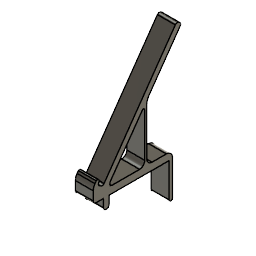
display-holder (Autodesk Fusion 360 design; units mm, degrees)
Autodesk Fusion 360 part; units mm, degrees
note: some values were not read from the file. Set by a fixed rule: which sketch regions a step uses.
(part 1 of 3)
sketch "Sketch1" plane through (0, 0, 0) normal (0, 1, 0) x (1, 0, 0) in component "breadboard"
  line L0 (0, 0) -> (83, 0)
  line L1 (83, 0) -> (83, -10)
  line L2 (83, -10) -> (0, -10)
  line L3 (0, -10) -> (0, 0)
  line L4 (13, 0) -> (17, 0)
  line L5 (17, 0) -> (17, -5)
  line L6 (17, -5) -> (13, -5)
  line L7 (13, -5) -> (13, 0)
  line L8 (66, 0) -> (70, 0)
  line L9 (70, 0) -> (70, -5)
  line L10 (70, -5) -> (66, -5)
  line L11 (66, -5) -> (66, 0)
  dimension "d1" = 10
  dimension "d2" = 83
  constraint horizontal L0
  constraint vertical L1
  constraint horizontal L2
  constraint vertical L3
  constraint coincident L0.start L3.end
  constraint horizontal L4
  constraint vertical L5
  constraint horizontal L6
  constraint vertical L7
  constraint horizontal L8
  constraint vertical L9
  constraint horizontal L10
  constraint vertical L11
  measures "d1" distance of L0.start L2.end
  measures "d2" distance of L0.start L0.end
extrude "Extrude3" add sketch "Sketch1" along normal blind 10 makes body 1 in component "breadboard"
extrude "Extrude5" add sketch "Sketch1" against normal blind 1 contours L0 L4 L5 L6 L7 | L0 L8 L9 L10 L11 bodies 1 in component "breadboard"
sketch "Sketch5" plane through (83, 0, 0) normal (1, 0, 0) x (0, 1, 0) in component "breadboard"
  line L0 (0, 10) -> (0, 0)
  line L1 (0, 0) -> (10, 0)
  line L2 (10, 0) -> (10, 10)
  line L3 (10, 10) -> (0, 10)
  line L4 (3, 0) -> (7, 0)
  line L5 (7, 0) -> (7, 5)
  line L6 (7, 5) -> (3, 5)
  line L7 (3, 5) -> (3, 0)
  constraint coincident L1 L4.start
  constraint horizontal L4
  constraint vertical L5
  constraint horizontal L6
  constraint vertical L7
extrude "Extrude6" add sketch "Sketch5" along normal blind 1 contours L1 L4 L5 L6 L7 bodies 1 in component "breadboard"
sketch "Sketch6" plane through (0, 0, 0) normal (-1, 0, 0) x (0, -1, 0) in component "breadboard"
  line L0 (0, 0) -> (0, 10)
  line L1 (0, 10) -> (-10, 10)
  line L2 (-10, 10) -> (-10, 0)
  line L3 (-10, 0) -> (0, 0)
  line L4 (-7, 0) -> (-3, 0)
  line L5 (-3, 0) -> (-3, 4)
  line L6 (-3, 4) -> (-7, 4)
  line L7 (-7, 4) -> (-7, 0)
  line L8 (-3, 5) -> (-3, 0)
  point P0 (-7, 0)
  constraint coincident P0 L4.start
  constraint horizontal L4
  constraint vertical L5
  constraint horizontal L6
  constraint vertical L7
  constraint coincident L5.end L8
extrude "Extrude7" cut sketch "Sketch6" against normal blind 1 contours L3 L4 L5 L6 L7 L8 bodies 1 in component "breadboard"
sketch "Sketch8" plane through (0, 0, 0) normal (0, 0, 1) x (1, 0, 0) in component "breadboard"
  line L0 (0, 45) -> (83, 45)
  line L1 (83, 45) -> (83, 10)
  line L2 (83, 10) -> (0, 10)
  line L3 (0, 10) -> (0, 45)
  point P0 (0, 45)
  point P1 (83, 10)
  constraint horizontal L0
  constraint vertical L1
  constraint horizontal L2
  constraint vertical L3
  constraint coincident P1 L1.end
  constraint coincident P0 L0.start
extrude "Extrude8" add sketch "Sketch8" along normal blind 10 separate body makes body 2 in component "breadboard"
sketch "Sketch9" plane through (0, 0, 10) normal (0, 0, 1) x (-1, 0, 0) in component "breadboard"
  line L0 (-83, -10) -> (-83, -45)
  line L1 (0, -45) -> (0, -10)
  line L2 (0, -26.5) -> (-83, -26.5)
  line L3 (0, -28.5) -> (-83, -28.5)
  line L4 (0, -10) -> (-83, -10)
  line L5 (-83, -45) -> (0, -45)
  line L6 (-5.0001, -15.25) -> (-5.0001, -17.25)
  line L7 (-5.0001, -17.25) -> (-3.0001, -17.25)
  line L8 (-3.0001, -17.25) -> (-3.0001, -15.25)
  line L9 (-3.0001, -15.25) -> (-5.0001, -15.25)
  line L10 (-3.0001, -17.75) -> (-5.0001, -17.75)
  line L11 (-5.0001, -17.75) -> (-5.0001, -19.75)
  line L12 (-5.0001, -19.75) -> (-3.0001, -19.75)
  line L13 (-3.0001, -19.75) -> (-3.0001, -17.75)
  line L14 (-5.0001, -22.25) -> (-3.0001, -22.25)
  line L15 (-3.0001, -22.25) -> (-3.0001, -20.25)
  line L16 (-3.0001, -20.25) -> (-5.0001, -20.25)
  line L17 (-5.0001, -20.25) -> (-5.0001, -22.25)
  line L18 (-5.0001, -24.75) -> (-3.0001, -24.75)
  line L19 (-3.0001, -24.75) -> (-3.0001, -22.75)
  line L20 (-5.0001, -22.75) -> (-5.0001, -24.75)
  line L21 (-3.0001, -22.75) -> (-5.0001, -22.75)
  line L22 (-5.0001, -14.75) -> (-3.0001, -14.75)
  line L23 (-3.0001, -14.75) -> (-3.0001, -12.75)
  line L24 (-3.0001, -12.75) -> (-5.0001, -12.75)
  line L25 (-5.0001, -12.75) -> (-5.0001, -14.75)
  line L26 (-7.5001, -15.25) -> (-7.5001, -17.25)
  line L27 (-5.5001, -24.75) -> (-5.5001, -22.75)
  line L28 (-5.5001, -22.75) -> (-7.5001, -22.75)
  line L29 (-5.5001, -17.25) -> (-5.5001, -15.25)
  line L30 (-7.5001, -14.75) -> (-5.5001, -14.75)
  line L31 (-7.5001, -12.75) -> (-7.5001, -14.75)
  line L32 (-5.5001, -15.25) -> (-7.5001, -15.25)
  line L33 (-7.5001, -17.25) -> (-5.5001, -17.25)
  line L34 (-7.5001, -22.75) -> (-7.5001, -24.75)
  line L35 (-5.5001, -22.25) -> (-5.5001, -20.25)
  line L36 (-5.5001, -12.75) -> (-7.5001, -12.75)
  line L37 (-5.5001, -20.25) -> (-7.5001, -20.25)
  line L38 (-7.5001, -22.25) -> (-5.5001, -22.25)
  line L39 (-5.5001, -17.75) -> (-7.5001, -17.75)
  line L40 (-5.5001, -19.75) -> (-5.5001, -17.75)
  line L41 (-7.5001, -19.75) -> (-5.5001, -19.75)
  line L42 (-7.5001, -20.25) -> (-7.5001, -22.25)
  line L43 (-7.5001, -17.75) -> (-7.5001, -19.75)
  line L44 (-5.5001, -14.75) -> (-5.5001, -12.75)
  line L45 (-7.5001, -24.75) -> (-5.5001, -24.75)
  line L46 (-12.5001, -15.25) -> (-12.5001, -17.25)
  line L47 (-8.0001, -22.25) -> (-8.0001, -20.25)
  line L48 (-10.5001, -22.25) -> (-10.5001, -20.25)
  line L49 (-10.5001, -15.25) -> (-12.5001, -15.25)
  line L50 (-10.5001, -20.25) -> (-12.5001, -20.25)
  line L51 (-8.0001, -20.25) -> (-10.0001, -20.25)
  line L52 (-10.5001, -14.75) -> (-10.5001, -12.75)
  line L53 (-12.5001, -12.75) -> (-12.5001, -14.75)
  line L54 (-12.5001, -20.25) -> (-12.5001, -22.25)
  line L55 (-8.0001, -12.75) -> (-10.0001, -12.75)
  line L56 (-10.5001, -19.75) -> (-10.5001, -17.75)
  line L57 (-10.5001, -17.25) -> (-10.5001, -15.25)
  line L58 (-10.0001, -22.25) -> (-8.0001, -22.25)
  line L59 (-12.5001, -19.75) -> (-10.5001, -19.75)
  line L60 (-8.0001, -15.25) -> (-10.0001, -15.25)
  line L61 (-10.0001, -15.25) -> (-10.0001, -17.25)
  line L62 (-8.0001, -22.75) -> (-10.0001, -22.75)
  line L63 (-10.0001, -24.75) -> (-8.0001, -24.75)
  line L64 (-8.0001, -19.75) -> (-8.0001, -17.75)
  line L65 (-10.0001, -20.25) -> (-10.0001, -22.25)
  line L66 (-8.0001, -17.75) -> (-10.0001, -17.75)
  line L67 (-12.5001, -17.75) -> (-12.5001, -19.75)
  line L68 (-10.0001, -22.75) -> (-10.0001, -24.75)
  line L69 (-10.5001, -17.75) -> (-12.5001, -17.75)
  line L70 (-10.5001, -12.75) -> (-12.5001, -12.75)
  line L71 (-8.0001, -24.75) -> (-8.0001, -22.75)
  line L72 (-10.0001, -17.75) -> (-10.0001, -19.75)
  line L73 (-10.0001, -12.75) -> (-10.0001, -14.75)
  line L74 (-12.5001, -14.75) -> (-10.5001, -14.75)
  line L75 (-12.5001, -24.75) -> (-10.5001, -24.75)
  line L76 (-12.5001, -22.25) -> (-10.5001, -22.25)
  line L77 (-10.5001, -22.75) -> (-12.5001, -22.75)
  line L78 (-10.0001, -14.75) -> (-8.0001, -14.75)
  line L79 (-8.0001, -14.75) -> (-8.0001, -12.75)
  line L80 (-12.5001, -17.25) -> (-10.5001, -17.25)
  line L81 (-8.0001, -17.25) -> (-8.0001, -15.25)
  line L82 (-10.5001, -24.75) -> (-10.5001, -22.75)
  line L83 (-12.5001, -22.75) -> (-12.5001, -24.75)
  line L84 (-10.0001, -17.25) -> (-8.0001, -17.25)
  line L85 (-10.0001, -19.75) -> (-8.0001, -19.75)
  line L86 (-13.0001, -17.25) -> (-13.0001, -15.25)
  line L87 (-17.5001, -17.75) -> (-17.5001, -19.75)
  line L88 (-15.0001, -12.75) -> (-15.0001, -14.75)
  line L89 (-13.0001, -15.25) -> (-15.0001, -15.25)
  line L90 (-15.5001, -17.25) -> (-15.5001, -15.25)
  line L91 (-15.0001, -22.25) -> (-13.0001, -22.25)
  line L92 (-15.5001, -24.75) -> (-15.5001, -22.75)
  line L93 (-18.0001, -19.75) -> (-18.0001, -17.75)
  line L94 (-15.5001, -22.75) -> (-17.5001, -22.75)
  line L95 (-13.0001, -22.75) -> (-15.0001, -22.75)
  line L96 (-13.0001, -14.75) -> (-13.0001, -12.75)
  line L97 (-15.5001, -14.75) -> (-15.5001, -12.75)
  line L98 (-15.5001, -19.75) -> (-15.5001, -17.75)
  line L99 (-15.0001, -14.75) -> (-13.0001, -14.75)
  line L100 (-13.0001, -24.75) -> (-13.0001, -22.75)
  line L101 (-13.0001, -12.75) -> (-15.0001, -12.75)
  line L102 (-15.0001, -17.25) -> (-13.0001, -17.25)
  line L103 (-15.0001, -24.75) -> (-13.0001, -24.75)
  line L104 (-17.5001, -20.25) -> (-17.5001, -22.25)
  line L105 (-18.0001, -15.25) -> (-20.0001, -15.25)
  line L106 (-18.0001, -12.75) -> (-20.0001, -12.75)
  line L107 (-17.5001, -12.75) -> (-17.5001, -14.75)
  line L108 (-15.0001, -20.25) -> (-15.0001, -22.25)
  line L109 (-15.0001, -19.75) -> (-13.0001, -19.75)
  line L110 (-18.0001, -17.25) -> (-18.0001, -15.25)
  line L111 (-20.0001, -14.75) -> (-18.0001, -14.75)
  line L112 (-22.5001, -20.25) -> (-22.5001, -22.25)
  line L113 (-20.0001, -12.75) -> (-20.0001, -14.75)
  line L114 (-18.0001, -14.75) -> (-18.0001, -12.75)
  line L115 (-20.5001, -20.25) -> (-22.5001, -20.25)
  line L116 (-20.5001, -22.75) -> (-22.5001, -22.75)
  line L117 (-22.5001, -12.75) -> (-22.5001, -14.75)
  line L118 (-20.5001, -17.25) -> (-20.5001, -15.25)
  line L119 (-20.0001, -15.25) -> (-20.0001, -17.25)
  line L120 (-20.5001, -15.25) -> (-22.5001, -15.25)
  line L121 (-22.5001, -15.25) -> (-22.5001, -17.25)
  line L122 (-17.5001, -15.25) -> (-17.5001, -17.25)
  line L123 (-15.5001, -22.25) -> (-15.5001, -20.25)
  line L124 (-20.0001, -20.25) -> (-20.0001, -22.25)
  line L125 (-18.0001, -22.25) -> (-18.0001, -20.25)
  line L126 (-13.0001, -22.25) -> (-13.0001, -20.25)
  line L127 (-22.5001, -19.75) -> (-20.5001, -19.75)
  line L128 (-22.5001, -17.25) -> (-20.5001, -17.25)
  line L129 (-22.5001, -14.75) -> (-20.5001, -14.75)
  line L130 (-20.5001, -12.75) -> (-22.5001, -12.75)
  line L131 (-20.0001, -17.25) -> (-18.0001, -17.25)
  line L132 (-20.0001, -17.75) -> (-20.0001, -19.75)
  line L133 (-15.5001, -20.25) -> (-17.5001, -20.25)
  line L134 (-15.5001, -12.75) -> (-17.5001, -12.75)
  line L135 (-20.0001, -22.75) -> (-20.0001, -24.75)
  line L136 (-20.5001, -17.75) -> (-22.5001, -17.75)
  line L137 (-20.0001, -24.75) -> (-18.0001, -24.75)
  line L138 (-22.5001, -17.75) -> (-22.5001, -19.75)
  line L139 (-18.0001, -22.75) -> (-20.0001, -22.75)
  line L140 (-20.0001, -22.25) -> (-18.0001, -22.25)
  line L141 (-20.5001, -19.75) -> (-20.5001, -17.75)
  line L142 (-18.0001, -24.75) -> (-18.0001, -22.75)
  line L143 (-17.5001, -22.75) -> (-17.5001, -24.75)
  line L144 (-20.5001, -14.75) -> (-20.5001, -12.75)
  line L145 (-13.0001, -20.25) -> (-15.0001, -20.25)
  line L146 (-13.0001, -19.75) -> (-13.0001, -17.75)
  line L147 (-17.5001, -17.25) -> (-15.5001, -17.25)
  line L148 (-17.5001, -19.75) -> (-15.5001, -19.75)
  line L149 (-18.0001, -20.25) -> (-20.0001, -20.25)
  line L150 (-15.5001, -17.75) -> (-17.5001, -17.75)
  line L151 (-15.0001, -15.25) -> (-15.0001, -17.25)
  line L152 (-15.0001, -22.75) -> (-15.0001, -24.75)
  line L153 (-17.5001, -14.75) -> (-15.5001, -14.75)
  line L154 (-18.0001, -17.75) -> (-20.0001, -17.75)
  line L155 (-13.0001, -17.75) -> (-15.0001, -17.75)
  line L156 (-15.5001, -15.25) -> (-17.5001, -15.25)
  line L157 (-22.5001, -22.25) -> (-20.5001, -22.25)
  line L158 (-22.5001, -22.75) -> (-22.5001, -24.75)
  line L159 (-20.5001, -22.25) -> (-20.5001, -20.25)
  line L160 (-17.5001, -24.75) -> (-15.5001, -24.75)
  line L161 (-20.5001, -24.75) -> (-20.5001, -22.75)
  line L162 (-20.0001, -19.75) -> (-18.0001, -19.75)
  line L163 (-17.5001, -22.25) -> (-15.5001, -22.25)
  line L164 (-15.0001, -17.75) -> (-15.0001, -19.75)
  line L165 (-22.5001, -24.75) -> (-20.5001, -24.75)
  line L166 (-40.5001, -19.75) -> (-40.5001, -17.75)
  line L167 (-38.0001, -20.25) -> (-40.0001, -20.25)
  line L168 (-42.5001, -17.25) -> (-40.5001, -17.25)
  line L169 (-37.5001, -17.75) -> (-37.5001, -19.75)
  line L170 (-40.5001, -17.75) -> (-42.5001, -17.75)
  line L171 (-40.0001, -17.75) -> (-40.0001, -19.75)
  line L172 (-40.5001, -20.25) -> (-42.5001, -20.25)
  line L173 (-40.0001, -17.25) -> (-38.0001, -17.25)
  line L174 (-40.0001, -19.75) -> (-38.0001, -19.75)
  line L175 (-35.5001, -17.75) -> (-37.5001, -17.75)
  line L176 (-35.5001, -20.25) -> (-37.5001, -20.25)
  line L177 (-37.5001, -19.75) -> (-35.5001, -19.75)
  line L178 (-37.5001, -17.25) -> (-35.5001, -17.25)
  line L179 (-42.5001, -19.75) -> (-40.5001, -19.75)
  line L180 (-38.0001, -17.75) -> (-40.0001, -17.75)
  line L181 (-35.5001, -19.75) -> (-35.5001, -17.75)
  line L182 (-38.0001, -19.75) -> (-38.0001, -17.75)
  line L183 (-42.5001, -17.75) -> (-42.5001, -19.75)
  line L184 (-42.5001, -22.75) -> (-42.5001, -24.75)
  line L185 (-38.0001, -22.75) -> (-40.0001, -22.75)
  line L186 (-35.5001, -22.25) -> (-35.5001, -20.25)
  line L187 (-27.5001, -20.25) -> (-27.5001, -22.25)
  line L188 (-35.5001, -12.75) -> (-37.5001, -12.75)
  line L189 (-40.0001, -20.25) -> (-40.0001, -22.25)
  line L190 (-42.5001, -22.25) -> (-40.5001, -22.25)
  line L191 (-37.5001, -14.75) -> (-35.5001, -14.75)
  line L192 (-35.5001, -22.75) -> (-37.5001, -22.75)
  line L193 (-40.5001, -12.75) -> (-42.5001, -12.75)
  line L194 (-25.0001, -17.25) -> (-23.0001, -17.25)
  line L195 (-37.5001, -24.75) -> (-35.5001, -24.75)
  line L196 (-37.5001, -20.25) -> (-37.5001, -22.25)
  line L197 (-25.0001, -24.75) -> (-23.0001, -24.75)
  line L198 (-35.5001, -15.25) -> (-37.5001, -15.25)
  line L199 (-38.0001, -24.75) -> (-38.0001, -22.75)
  line L200 (-40.0001, -22.25) -> (-38.0001, -22.25)
  line L201 (-42.5001, -24.75) -> (-40.5001, -24.75)
  line L202 (-42.5001, -20.25) -> (-42.5001, -22.25)
  line L203 (-40.5001, -15.25) -> (-42.5001, -15.25)
  line L204 (-40.0001, -24.75) -> (-38.0001, -24.75)
  line L205 (-40.5001, -24.75) -> (-40.5001, -22.75)
  line L206 (-38.0001, -22.25) -> (-38.0001, -20.25)
  line L207 (-42.5001, -14.75) -> (-40.5001, -14.75)
  line L208 (-40.0001, -15.25) -> (-40.0001, -17.25)
  line L209 (-38.0001, -17.25) -> (-38.0001, -15.25)
  line L210 (-37.5001, -22.75) -> (-37.5001, -24.75)
  line L211 (-40.5001, -22.75) -> (-42.5001, -22.75)
  line L212 (-40.5001, -17.25) -> (-40.5001, -15.25)
  line L213 (-37.5001, -22.25) -> (-35.5001, -22.25)
  line L214 (-25.0001, -19.75) -> (-23.0001, -19.75)
  line L215 (-42.5001, -15.25) -> (-42.5001, -17.25)
  line L216 (-32.5001, -20.25) -> (-32.5001, -22.25)
  line L217 (-37.5001, -15.25) -> (-37.5001, -17.25)
  line L218 (-40.5001, -22.25) -> (-40.5001, -20.25)
  line L219 (-40.0001, -22.75) -> (-40.0001, -24.75)
  line L220 (-32.5001, -17.75) -> (-32.5001, -19.75)
  line L221 (-35.0001, -17.75) -> (-35.0001, -19.75)
  line L222 (-28.0001, -22.75) -> (-30.0001, -22.75)
  line L223 (-40.0001, -14.75) -> (-38.0001, -14.75)
  line L224 (-38.0001, -15.25) -> (-40.0001, -15.25)
  line L225 (-27.5001, -17.75) -> (-27.5001, -19.75)
  line L226 (-27.5001, -24.75) -> (-25.5001, -24.75)
  line L227 (-32.5001, -15.25) -> (-32.5001, -17.25)
  line L228 (-33.0001, -20.25) -> (-35.0001, -20.25)
  line L229 (-35.0001, -17.25) -> (-33.0001, -17.25)
  line L230 (-25.5001, -15.25) -> (-27.5001, -15.25)
  line L231 (-27.5001, -22.75) -> (-27.5001, -24.75)
  line L232 (-35.5001, -24.75) -> (-35.5001, -22.75)
  line L233 (-25.0001, -20.25) -> (-25.0001, -22.25)
  line L234 (-35.0001, -19.75) -> (-33.0001, -19.75)
  line L235 (-40.5001, -14.75) -> (-40.5001, -12.75)
  line L236 (-30.5001, -17.25) -> (-30.5001, -15.25)
  line L237 (-30.0001, -17.75) -> (-30.0001, -19.75)
  line L238 (-30.0001, -22.75) -> (-30.0001, -24.75)
  line L239 (-25.5001, -22.75) -> (-27.5001, -22.75)
  line L240 (-28.0001, -19.75) -> (-28.0001, -17.75)
  line L241 (-30.0001, -20.25) -> (-30.0001, -22.25)
  line L242 (-37.5001, -12.75) -> (-37.5001, -14.75)
  line L243 (-30.5001, -20.25) -> (-32.5001, -20.25)
  line L244 (-27.5001, -17.25) -> (-25.5001, -17.25)
  line L245 (-32.5001, -24.75) -> (-30.5001, -24.75)
  line L246 (-25.5001, -12.75) -> (-27.5001, -12.75)
  line L247 (-25.0001, -17.75) -> (-25.0001, -19.75)
  line L248 (-23.0001, -22.25) -> (-23.0001, -20.25)
  line L249 (-32.5001, -22.25) -> (-30.5001, -22.25)
  line L250 (-30.5001, -19.75) -> (-30.5001, -17.75)
  line L251 (-28.0001, -20.25) -> (-30.0001, -20.25)
  line L252 (-32.5001, -19.75) -> (-30.5001, -19.75)
  line L253 (-35.0001, -15.25) -> (-35.0001, -17.25)
  line L254 (-35.5001, -17.25) -> (-35.5001, -15.25)
  line L255 (-33.0001, -17.25) -> (-33.0001, -15.25)
  line L256 (-42.5001, -12.75) -> (-42.5001, -14.75)
  line L257 (-38.0001, -12.75) -> (-40.0001, -12.75)
  line L258 (-30.5001, -17.75) -> (-32.5001, -17.75)
  line L259 (-25.5001, -22.25) -> (-25.5001, -20.25)
  line L260 (-33.0001, -19.75) -> (-33.0001, -17.75)
  line L261 (-30.0001, -22.25) -> (-28.0001, -22.25)
  line L262 (-30.0001, -19.75) -> (-28.0001, -19.75)
  line L263 (-28.0001, -24.75) -> (-28.0001, -22.75)
  line L264 (-30.0001, -24.75) -> (-28.0001, -24.75)
  line L265 (-25.5001, -17.75) -> (-27.5001, -17.75)
  line L266 (-23.0001, -20.25) -> (-25.0001, -20.25)
  line L267 (-33.0001, -17.75) -> (-35.0001, -17.75)
  line L268 (-32.5001, -22.75) -> (-32.5001, -24.75)
  line L269 (-28.0001, -22.25) -> (-28.0001, -20.25)
  line L270 (-27.5001, -22.25) -> (-25.5001, -22.25)
  line L271 (-30.5001, -22.75) -> (-32.5001, -22.75)
  line L272 (-40.0001, -12.75) -> (-40.0001, -14.75)
  line L273 (-38.0001, -14.75) -> (-38.0001, -12.75)
  line L274 (-28.0001, -17.75) -> (-30.0001, -17.75)
  line L275 (-30.5001, -12.75) -> (-32.5001, -12.75)
  line L276 (-30.5001, -14.75) -> (-30.5001, -12.75)
  line L277 (-30.5001, -15.25) -> (-32.5001, -15.25)
  line L278 (-27.5001, -12.75) -> (-27.5001, -14.75)
  line L279 (-33.0001, -15.25) -> (-35.0001, -15.25)
  line L280 (-30.0001, -17.25) -> (-28.0001, -17.25)
  line L281 (-30.0001, -15.25) -> (-30.0001, -17.25)
  line L282 (-27.5001, -15.25) -> (-27.5001, -17.25)
  line L283 (-25.0001, -22.25) -> (-23.0001, -22.25)
  line L284 (-23.0001, -19.75) -> (-23.0001, -17.75)
  line L285 (-33.0001, -12.75) -> (-35.0001, -12.75)
  line L286 (-35.0001, -12.75) -> (-35.0001, -14.75)
  line L287 (-28.0001, -12.75) -> (-30.0001, -12.75)
  line L288 (-25.5001, -24.75) -> (-25.5001, -22.75)
  line L289 (-27.5001, -14.75) -> (-25.5001, -14.75)
  line L290 (-25.0001, -22.75) -> (-25.0001, -24.75)
  line L291 (-28.0001, -17.25) -> (-28.0001, -15.25)
  line L292 (-35.0001, -14.75) -> (-33.0001, -14.75)
  line L293 (-25.5001, -19.75) -> (-25.5001, -17.75)
  line L294 (-30.0001, -14.75) -> (-28.0001, -14.75)
  line L295 (-25.0001, -14.75) -> (-23.0001, -14.75)
  line L296 (-33.0001, -22.25) -> (-33.0001, -20.25)
  line L297 (-25.5001, -20.25) -> (-27.5001, -20.25)
  line L298 (-28.0001, -15.25) -> (-30.0001, -15.25)
  line L299 (-32.5001, -17.25) -> (-30.5001, -17.25)
  line L300 (-35.0001, -22.25) -> (-33.0001, -22.25)
  line L301 (-35.0001, -22.75) -> (-35.0001, -24.75)
  line L302 (-23.0001, -17.75) -> (-25.0001, -17.75)
  line L303 (-35.0001, -20.25) -> (-35.0001, -22.25)
  line L304 (-35.5001, -14.75) -> (-35.5001, -12.75)
  line L305 (-30.0001, -12.75) -> (-30.0001, -14.75)
  line L306 (-23.0001, -22.75) -> (-25.0001, -22.75)
  line L307 (-32.5001, -12.75) -> (-32.5001, -14.75)
  line L308 (-27.5001, -19.75) -> (-25.5001, -19.75)
  line L309 (-23.0001, -24.75) -> (-23.0001, -22.75)
  line L310 (-28.0001, -14.75) -> (-28.0001, -12.75)
  line L311 (-33.0001, -14.75) -> (-33.0001, -12.75)
  line L312 (-32.5001, -14.75) -> (-30.5001, -14.75)
  line L313 (-25.5001, -14.75) -> (-25.5001, -12.75)
  line L314 (-33.0001, -22.75) -> (-35.0001, -22.75)
  line L315 (-33.0001, -24.75) -> (-33.0001, -22.75)
  line L316 (-23.0001, -14.75) -> (-23.0001, -12.75)
  line L317 (-23.0001, -17.25) -> (-23.0001, -15.25)
  line L318 (-35.0001, -24.75) -> (-33.0001, -24.75)
  line L319 (-23.0001, -12.75) -> (-25.0001, -12.75)
  line L320 (-23.0001, -15.25) -> (-25.0001, -15.25)
  line L321 (-30.5001, -24.75) -> (-30.5001, -22.75)
  line L322 (-30.5001, -22.25) -> (-30.5001, -20.25)
  line L323 (-25.0001, -15.25) -> (-25.0001, -17.25)
  line L324 (-25.5001, -17.25) -> (-25.5001, -15.25)
  line L325 (-25.0001, -12.75) -> (-25.0001, -14.75)
  line L326 (-73.0001, -17.75) -> (-75.0001, -17.75)
  line L327 (-77.5001, -14.75) -> (-75.5001, -14.75)
  line L328 (-73.0001, -12.75) -> (-75.0001, -12.75)
  line L329 (-75.0001, -12.75) -> (-75.0001, -14.75)
  line L330 (-73.0001, -14.75) -> (-73.0001, -12.75)
  line L331 (-75.5001, -17.75) -> (-77.5001, -17.75)
  line L332 (-75.0001, -14.75) -> (-73.0001, -14.75)
  line L333 (-72.5001, -15.25) -> (-72.5001, -17.25)
  line L334 (-73.0001, -15.25) -> (-75.0001, -15.25)
  line L335 (-75.0001, -17.25) -> (-73.0001, -17.25)
  line L336 (-72.5001, -12.75) -> (-72.5001, -14.75)
  line L337 (-73.0001, -17.25) -> (-73.0001, -15.25)
  line L338 (-77.5001, -15.25) -> (-77.5001, -17.25)
  line L339 (-78.0001, -14.75) -> (-78.0001, -12.75)
  line L340 (-78.0001, -17.25) -> (-78.0001, -15.25)
  line L341 (-75.5001, -12.75) -> (-77.5001, -12.75)
  line L342 (-77.5001, -12.75) -> (-77.5001, -14.75)
  line L343 (-75.5001, -14.75) -> (-75.5001, -12.75)
  line L344 (-75.5001, -15.25) -> (-77.5001, -15.25)
  line L345 (-75.5001, -17.25) -> (-75.5001, -15.25)
  line L346 (-77.5001, -17.25) -> (-75.5001, -17.25)
  line L347 (-65.5001, -24.75) -> (-65.5001, -22.75)
  line L348 (-67.5001, -22.25) -> (-65.5001, -22.25)
  line L349 (-67.5001, -19.75) -> (-65.5001, -19.75)
  line L350 (-65.0001, -20.25) -> (-65.0001, -22.25)
  line L351 (-67.5001, -17.25) -> (-65.5001, -17.25)
  line L352 (-65.5001, -20.25) -> (-67.5001, -20.25)
  line L353 (-65.5001, -19.75) -> (-65.5001, -17.75)
  line L354 (-65.0001, -17.75) -> (-65.0001, -19.75)
  line L355 (-65.0001, -22.75) -> (-65.0001, -24.75)
  line L356 (-67.5001, -24.75) -> (-65.5001, -24.75)
  line L357 (-65.5001, -22.75) -> (-67.5001, -22.75)
  line L358 (-65.5001, -17.75) -> (-67.5001, -17.75)
  line L359 (-63.0001, -12.75) -> (-65.0001, -12.75)
  line L360 (-52.5001, -24.75) -> (-50.5001, -24.75)
  line L361 (-52.5001, -20.25) -> (-52.5001, -22.25)
  line L362 (-45.0001, -24.75) -> (-43.0001, -24.75)
  line L363 (-63.0001, -22.75) -> (-65.0001, -22.75)
  line L364 (-65.0001, -17.25) -> (-63.0001, -17.25)
  line L365 (-73.0001, -20.25) -> (-75.0001, -20.25)
  line L366 (-75.5001, -22.25) -> (-75.5001, -20.25)
  line L367 (-65.0001, -14.75) -> (-63.0001, -14.75)
  line L368 (-72.5001, -17.75) -> (-72.5001, -19.75)
  line L369 (-65.0001, -19.75) -> (-63.0001, -19.75)
  line L370 (-47.5001, -20.25) -> (-47.5001, -22.25)
  line L371 (-65.0001, -22.25) -> (-63.0001, -22.25)
  line L372 (-75.0001, -19.75) -> (-73.0001, -19.75)
  line L373 (-75.0001, -22.25) -> (-73.0001, -22.25)
  line L374 (-45.0001, -19.75) -> (-43.0001, -19.75)
  line L375 (-78.0001, -22.25) -> (-78.0001, -20.25)
  line L376 (-63.0001, -15.25) -> (-65.0001, -15.25)
  line L377 (-75.0001, -20.25) -> (-75.0001, -22.25)
  line L378 (-77.5001, -22.25) -> (-75.5001, -22.25)
  line L379 (-77.5001, -19.75) -> (-75.5001, -19.75)
  line L380 (-63.0001, -20.25) -> (-65.0001, -20.25)
  line L381 (-75.5001, -20.25) -> (-77.5001, -20.25)
  line L382 (-65.0001, -24.75) -> (-63.0001, -24.75)
  line L383 (-77.5001, -20.25) -> (-77.5001, -22.25)
  line L384 (-73.0001, -19.75) -> (-73.0001, -17.75)
  line L385 (-72.5001, -20.25) -> (-72.5001, -22.25)
  line L386 (-60.5001, -12.75) -> (-62.5001, -12.75)
  line L387 (-75.0001, -24.75) -> (-73.0001, -24.75)
  line L388 (-60.5001, -15.25) -> (-62.5001, -15.25)
  line L389 (-43.0001, -22.25) -> (-43.0001, -20.25)
  line L390 (-72.5001, -22.75) -> (-72.5001, -24.75)
  line L391 (-68.0001, -17.75) -> (-70.0001, -17.75)
  line L392 (-50.0001, -12.75) -> (-50.0001, -14.75)
  line L393 (-48.0001, -12.75) -> (-50.0001, -12.75)
  line L394 (-62.5001, -22.25) -> (-60.5001, -22.25)
  line L395 (-45.5001, -12.75) -> (-47.5001, -12.75)
  line L396 (-78.0001, -20.25) -> (-80.0001, -20.25)
  line L397 (-45.0001, -20.25) -> (-45.0001, -22.25)
  line L398 (-50.5001, -15.25) -> (-52.5001, -15.25)
  line L399 (-70.0001, -15.25) -> (-70.0001, -17.25)
  line L400 (-55.0001, -14.75) -> (-53.0001, -14.75)
  line L401 (-55.0001, -12.75) -> (-55.0001, -14.75)
  line L402 (-77.5001, -24.75) -> (-75.5001, -24.75)
  line L403 (-62.5001, -22.75) -> (-62.5001, -24.75)
  line L404 (-53.0001, -14.75) -> (-53.0001, -12.75)
  line L405 (-53.0001, -15.25) -> (-55.0001, -15.25)
  line L406 (-75.5001, -22.75) -> (-77.5001, -22.75)
  line L407 (-62.5001, -24.75) -> (-60.5001, -24.75)
  line L408 (-62.5001, -20.25) -> (-62.5001, -22.25)
  line L409 (-77.5001, -22.75) -> (-77.5001, -24.75)
  line L410 (-75.0001, -22.75) -> (-75.0001, -24.75)
  line L411 (-75.5001, -24.75) -> (-75.5001, -22.75)
  line L412 (-78.0001, -24.75) -> (-78.0001, -22.75)
  line L413 (-70.0001, -19.75) -> (-68.0001, -19.75)
  line L414 (-60.5001, -22.75) -> (-62.5001, -22.75)
  line L415 (-52.5001, -14.75) -> (-50.5001, -14.75)
  line L416 (-50.0001, -20.25) -> (-50.0001, -22.25)
  line L417 (-52.5001, -22.25) -> (-50.5001, -22.25)
  line L418 (-68.0001, -15.25) -> (-70.0001, -15.25)
  line L419 (-68.0001, -12.75) -> (-70.0001, -12.75)
  line L420 (-52.5001, -12.75) -> (-52.5001, -14.75)
  line L421 (-62.5001, -12.75) -> (-62.5001, -14.75)
  line L422 (-62.5001, -19.75) -> (-60.5001, -19.75)
  line L423 (-70.0001, -14.75) -> (-68.0001, -14.75)
  line L424 (-55.5001, -14.75) -> (-55.5001, -12.75)
  line L425 (-63.0001, -19.75) -> (-63.0001, -17.75)
  line L426 (-63.0001, -17.25) -> (-63.0001, -15.25)
  line L427 (-62.5001, -15.25) -> (-62.5001, -17.25)
  line L428 (-73.0001, -24.75) -> (-73.0001, -22.75)
  line L429 (-70.0001, -24.75) -> (-68.0001, -24.75)
  line L430 (-62.5001, -14.75) -> (-60.5001, -14.75)
  line L431 (-60.5001, -20.25) -> (-62.5001, -20.25)
  line L432 (-63.0001, -14.75) -> (-63.0001, -12.75)
  line L433 (-50.5001, -14.75) -> (-50.5001, -12.75)
  line L434 (-62.5001, -17.25) -> (-60.5001, -17.25)
  line L435 (-70.0001, -12.75) -> (-70.0001, -14.75)
  line L436 (-62.5001, -17.75) -> (-62.5001, -19.75)
  line L437 (-73.0001, -22.75) -> (-75.0001, -22.75)
  line L438 (-53.0001, -12.75) -> (-55.0001, -12.75)
  line L439 (-60.5001, -17.75) -> (-62.5001, -17.75)
  line L440 (-63.0001, -22.25) -> (-63.0001, -20.25)
  line L441 (-50.5001, -17.75) -> (-52.5001, -17.75)
  line L442 (-48.0001, -22.25) -> (-48.0001, -20.25)
  line L443 (-63.0001, -24.75) -> (-63.0001, -22.75)
  line L444 (-50.5001, -12.75) -> (-52.5001, -12.75)
  line L445 (-70.0001, -17.25) -> (-68.0001, -17.25)
  line L446 (-52.5001, -19.75) -> (-50.5001, -19.75)
  line L447 (-68.0001, -22.75) -> (-70.0001, -22.75)
  line L448 (-60.0001, -12.75) -> (-60.0001, -14.75)
  line L449 (-53.0001, -19.75) -> (-53.0001, -17.75)
  line L450 (-50.5001, -17.25) -> (-50.5001, -15.25)
  line L451 (-78.0001, -19.75) -> (-78.0001, -17.75)
  line L452 (-47.5001, -14.75) -> (-45.5001, -14.75)
  line L453 (-47.5001, -17.25) -> (-45.5001, -17.25)
  line L454 (-50.0001, -15.25) -> (-50.0001, -17.25)
  line L455 (-50.0001, -17.25) -> (-48.0001, -17.25)
  line L456 (-45.5001, -17.75) -> (-47.5001, -17.75)
  line L457 (-43.0001, -14.75) -> (-43.0001, -12.75)
  line L458 (-45.0001, -15.25) -> (-45.0001, -17.25)
  line L459 (-52.5001, -15.25) -> (-52.5001, -17.25)
  line L460 (-70.5001, -17.25) -> (-70.5001, -15.25)
  line L461 (-58.0001, -12.75) -> (-60.0001, -12.75)
  line L462 (-75.0001, -17.75) -> (-75.0001, -19.75)
  line L463 (-75.5001, -19.75) -> (-75.5001, -17.75)
  line L464 (-50.0001, -24.75) -> (-48.0001, -24.75)
  line L465 (-58.0001, -14.75) -> (-58.0001, -12.75)
  line L466 (-47.5001, -22.75) -> (-47.5001, -24.75)
  line L467 (-53.0001, -17.75) -> (-55.0001, -17.75)
  line L468 (-60.5001, -14.75) -> (-60.5001, -12.75)
  line L469 (-78.0001, -15.25) -> (-80.0001, -15.25)
  line L470 (-45.0001, -12.75) -> (-45.0001, -14.75)
  line L471 (-52.5001, -17.25) -> (-50.5001, -17.25)
  line L472 (-48.0001, -22.75) -> (-50.0001, -22.75)
  line L473 (-55.0001, -17.75) -> (-55.0001, -19.75)
  line L474 (-60.0001, -15.25) -> (-60.0001, -17.25)
  line L475 (-47.5001, -12.75) -> (-47.5001, -14.75)
  line L476 (-50.0001, -14.75) -> (-48.0001, -14.75)
  line L477 (-58.0001, -17.25) -> (-58.0001, -15.25)
  line L478 (-43.0001, -15.25) -> (-45.0001, -15.25)
  line L479 (-45.5001, -17.25) -> (-45.5001, -15.25)
  line L480 (-45.5001, -22.25) -> (-45.5001, -20.25)
  line L481 (-48.0001, -17.25) -> (-48.0001, -15.25)
  line L482 (-45.0001, -14.75) -> (-43.0001, -14.75)
  line L483 (-48.0001, -24.75) -> (-48.0001, -22.75)
  line L484 (-72.5001, -17.25) -> (-70.5001, -17.25)
  line L485 (-48.0001, -14.75) -> (-48.0001, -12.75)
  line L486 (-80.0001, -24.75) -> (-78.0001, -24.75)
  line L487 (-70.5001, -17.75) -> (-72.5001, -17.75)
  line L488 (-68.0001, -20.25) -> (-70.0001, -20.25)
  line L489 (-53.0001, -17.25) -> (-53.0001, -15.25)
  line L490 (-48.0001, -15.25) -> (-50.0001, -15.25)
  line L491 (-45.5001, -14.75) -> (-45.5001, -12.75)
  line L492 (-77.5001, -17.75) -> (-77.5001, -19.75)
  line L493 (-70.5001, -15.25) -> (-72.5001, -15.25)
  line L494 (-80.0001, -17.25) -> (-78.0001, -17.25)
  line L495 (-43.0001, -17.25) -> (-43.0001, -15.25)
  line L496 (-43.0001, -12.75) -> (-45.0001, -12.75)
  line L497 (-57.5001, -12.75) -> (-57.5001, -14.75)
  line L498 (-43.0001, -17.75) -> (-45.0001, -17.75)
  line L499 (-57.5001, -15.25) -> (-57.5001, -17.25)
  line L500 (-70.5001, -14.75) -> (-70.5001, -12.75)
  line L501 (-48.0001, -17.75) -> (-50.0001, -17.75)
  line L502 (-60.0001, -14.75) -> (-58.0001, -14.75)
  line L503 (-55.0001, -17.25) -> (-53.0001, -17.25)
  line L504 (-47.5001, -15.25) -> (-47.5001, -17.25)
  line L505 (-72.5001, -14.75) -> (-70.5001, -14.75)
  line L506 (-45.5001, -15.25) -> (-47.5001, -15.25)
  line L507 (-52.5001, -17.75) -> (-52.5001, -19.75)
  line L508 (-70.5001, -12.75) -> (-72.5001, -12.75)
  line L509 (-50.0001, -22.25) -> (-48.0001, -22.25)
  line L510 (-50.0001, -22.75) -> (-50.0001, -24.75)
  line L511 (-67.5001, -12.75) -> (-67.5001, -14.75)
  line L512 (-53.0001, -22.75) -> (-55.0001, -22.75)
  line L513 (-67.5001, -15.25) -> (-67.5001, -17.25)
  line L514 (-58.0001, -20.25) -> (-60.0001, -20.25)
  line L515 (-58.0001, -19.75) -> (-58.0001, -17.75)
  line L516 (-50.0001, -17.75) -> (-50.0001, -19.75)
  line L517 (-50.0001, -19.75) -> (-48.0001, -19.75)
  line L518 (-58.0001, -17.75) -> (-60.0001, -17.75)
  line L519 (-57.5001, -17.75) -> (-57.5001, -19.75)
  line L520 (-52.5001, -22.75) -> (-52.5001, -24.75)
  line L521 (-68.0001, -14.75) -> (-68.0001, -12.75)
  line L522 (-48.0001, -19.75) -> (-48.0001, -17.75)
  line L523 (-50.5001, -22.75) -> (-52.5001, -22.75)
  line L524 (-43.0001, -22.75) -> (-45.0001, -22.75)
  line L525 (-45.0001, -17.75) -> (-45.0001, -19.75)
  line L526 (-60.5001, -19.75) -> (-60.5001, -17.75)
  line L527 (-80.0001, -15.25) -> (-80.0001, -17.25)
  line L528 (-55.5001, -22.25) -> (-55.5001, -20.25)
  line L529 (-78.0001, -12.75) -> (-80.0001, -12.75)
  line L530 (-47.5001, -17.75) -> (-47.5001, -19.75)
  line L531 (-55.0001, -20.25) -> (-55.0001, -22.25)
  line L532 (-45.5001, -22.75) -> (-47.5001, -22.75)
  line L533 (-60.0001, -17.25) -> (-58.0001, -17.25)
  line L534 (-70.5001, -22.25) -> (-70.5001, -20.25)
  line L535 (-80.0001, -14.75) -> (-78.0001, -14.75)
  line L536 (-45.5001, -24.75) -> (-45.5001, -22.75)
  line L537 (-55.0001, -24.75) -> (-53.0001, -24.75)
  line L538 (-55.5001, -19.75) -> (-55.5001, -17.75)
  line L539 (-68.0001, -17.25) -> (-68.0001, -15.25)
  line L540 (-47.5001, -22.25) -> (-45.5001, -22.25)
  line L541 (-45.0001, -22.25) -> (-43.0001, -22.25)
  line L542 (-55.0001, -22.75) -> (-55.0001, -24.75)
  line L543 (-55.0001, -19.75) -> (-53.0001, -19.75)
  line L544 (-50.5001, -24.75) -> (-50.5001, -22.75)
  line L545 (-50.5001, -19.75) -> (-50.5001, -17.75)
  line L546 (-45.5001, -20.25) -> (-47.5001, -20.25)
  line L547 (-48.0001, -20.25) -> (-50.0001, -20.25)
  line L548 (-50.5001, -22.25) -> (-50.5001, -20.25)
  line L549 (-58.0001, -15.25) -> (-60.0001, -15.25)
  line L550 (-55.0001, -22.25) -> (-53.0001, -22.25)
  line L551 (-47.5001, -19.75) -> (-45.5001, -19.75)
  line L552 (-72.5001, -19.75) -> (-70.5001, -19.75)
  line L553 (-72.5001, -22.25) -> (-70.5001, -22.25)
  line L554 (-80.0001, -12.75) -> (-80.0001, -14.75)
  line L555 (-60.0001, -17.75) -> (-60.0001, -19.75)
  line L556 (-45.5001, -19.75) -> (-45.5001, -17.75)
  line L557 (-47.5001, -24.75) -> (-45.5001, -24.75)
  line L558 (-53.0001, -20.25) -> (-55.0001, -20.25)
  line L559 (-43.0001, -20.25) -> (-45.0001, -20.25)
  line L560 (-60.0001, -19.75) -> (-58.0001, -19.75)
  line L561 (-53.0001, -24.75) -> (-53.0001, -22.75)
  line L562 (-53.0001, -22.25) -> (-53.0001, -20.25)
  line L563 (-70.0001, -20.25) -> (-70.0001, -22.25)
  line L564 (-45.0001, -22.75) -> (-45.0001, -24.75)
  line L565 (-43.0001, -24.75) -> (-43.0001, -22.75)
  line L566 (-55.5001, -24.75) -> (-55.5001, -22.75)
  line L567 (-70.5001, -20.25) -> (-72.5001, -20.25)
  line L568 (-65.0001, -15.25) -> (-65.0001, -17.25)
  line L569 (-60.0001, -22.75) -> (-60.0001, -24.75)
  line L570 (-70.5001, -19.75) -> (-70.5001, -17.75)
  line L571 (-67.5001, -22.75) -> (-67.5001, -24.75)
  line L572 (-60.5001, -24.75) -> (-60.5001, -22.75)
  line L573 (-57.5001, -22.75) -> (-57.5001, -24.75)
  line L574 (-80.0001, -22.25) -> (-78.0001, -22.25)
  line L575 (-65.5001, -22.25) -> (-65.5001, -20.25)
  line L576 (-68.0001, -19.75) -> (-68.0001, -17.75)
  line L577 (-67.5001, -20.25) -> (-67.5001, -22.25)
  line L578 (-43.0001, -19.75) -> (-43.0001, -17.75)
  line L579 (-60.5001, -17.25) -> (-60.5001, -15.25)
  line L580 (-58.0001, -22.25) -> (-58.0001, -20.25)
  line L581 (-58.0001, -22.75) -> (-60.0001, -22.75)
  line L582 (-68.0001, -22.25) -> (-68.0001, -20.25)
  line L583 (-58.0001, -24.75) -> (-58.0001, -22.75)
  line L584 (-55.5001, -17.25) -> (-55.5001, -15.25)
  line L585 (-67.5001, -17.75) -> (-67.5001, -19.75)
  line L586 (-72.5001, -24.75) -> (-70.5001, -24.75)
  line L587 (-65.5001, -12.75) -> (-67.5001, -12.75)
  line L588 (-78.0001, -22.75) -> (-80.0001, -22.75)
  line L589 (-65.5001, -14.75) -> (-65.5001, -12.75)
  line L590 (-80.0001, -20.25) -> (-80.0001, -22.25)
  line L591 (-55.0001, -15.25) -> (-55.0001, -17.25)
  line L592 (-65.0001, -12.75) -> (-65.0001, -14.75)
  line L593 (-60.0001, -22.25) -> (-58.0001, -22.25)
  line L594 (-67.5001, -14.75) -> (-65.5001, -14.75)
  line L595 (-65.5001, -15.25) -> (-67.5001, -15.25)
  line L596 (-80.0001, -22.75) -> (-80.0001, -24.75)
  line L597 (-78.0001, -17.75) -> (-80.0001, -17.75)
  line L598 (-70.5001, -24.75) -> (-70.5001, -22.75)
  line L599 (-60.5001, -22.25) -> (-60.5001, -20.25)
  line L600 (-70.0001, -22.25) -> (-68.0001, -22.25)
  line L601 (-80.0001, -19.75) -> (-78.0001, -19.75)
  line L602 (-57.5001, -20.25) -> (-57.5001, -22.25)
  line L603 (-60.0001, -24.75) -> (-58.0001, -24.75)
  line L604 (-68.0001, -24.75) -> (-68.0001, -22.75)
  line L605 (-65.5001, -17.25) -> (-65.5001, -15.25)
  line L606 (-80.0001, -17.75) -> (-80.0001, -19.75)
  line L607 (-60.0001, -20.25) -> (-60.0001, -22.25)
  line L608 (-70.0001, -22.75) -> (-70.0001, -24.75)
  line L609 (-50.5001, -20.25) -> (-52.5001, -20.25)
  line L610 (-70.0001, -17.75) -> (-70.0001, -19.75)
  line L611 (-70.5001, -22.75) -> (-72.5001, -22.75)
  line L612 (-75.0001, -15.25) -> (-75.0001, -17.25)
  line L613 (-55.5001, -20.25) -> (-57.5001, -20.25)
  line L614 (-57.5001, -14.75) -> (-55.5001, -14.75)
  line L615 (-55.5001, -17.75) -> (-57.5001, -17.75)
  line L616 (-57.5001, -17.25) -> (-55.5001, -17.25)
  line L617 (-55.5001, -15.25) -> (-57.5001, -15.25)
  line L618 (-57.5001, -24.75) -> (-55.5001, -24.75)
  line L619 (-55.5001, -22.75) -> (-57.5001, -22.75)
  line L620 (-57.5001, -19.75) -> (-55.5001, -19.75)
  line L621 (-57.5001, -22.25) -> (-55.5001, -22.25)
  line L622 (-55.5001, -12.75) -> (-57.5001, -12.75)
  line L623 (-73.0001, -22.25) -> (-73.0001, -20.25)
  line L624 (-45.0001, -17.25) -> (-43.0001, -17.25)
  line L625 (-63.0001, -17.75) -> (-65.0001, -17.75)
  line L626 (-48.0001, -42.25) -> (-48.0001, -40.25)
  line L627 (-50.0001, -39.75) -> (-48.0001, -39.75)
  line L628 (-42.5001, -40.25) -> (-42.5001, -42.25)
  line L629 (-50.5001, -42.25) -> (-50.5001, -40.25)
  line L630 (-45.0001, -42.25) -> (-43.0001, -42.25)
  line L631 (-45.5001, -40.25) -> (-47.5001, -40.25)
  line L632 (-8.0001, -39.75) -> (-8.0001, -37.75)
  line L633 (-7.5001, -42.25) -> (-5.5001, -42.25)
  line L634 (-25.0001, -37.25) -> (-23.0001, -37.25)
  line L635 (-23.0001, -37.75) -> (-25.0001, -37.75)
  line L636 (-5.0001, -37.75) -> (-5.0001, -39.75)
  line L637 (-5.0001, -34.75) -> (-3.0001, -34.75)
  line L638 (-5.5001, -42.25) -> (-5.5001, -40.25)
  line L639 (-3.0001, -37.75) -> (-5.0001, -37.75)
  line L640 (-8.0001, -42.25) -> (-8.0001, -40.25)
  line L641 (-25.0001, -39.75) -> (-23.0001, -39.75)
  line L642 (-25.0001, -32.25) -> (-23.0001, -32.25)
  line L643 (-10.5001, -37.25) -> (-10.5001, -35.25)
  line L644 (-23.0001, -35.25) -> (-25.0001, -35.25)
  line L645 (-7.5001, -37.25) -> (-5.5001, -37.25)
  line L646 (-17.5001, -34.75) -> (-15.5001, -34.75)
  line L647 (-10.0001, -42.25) -> (-8.0001, -42.25)
  line L648 (-5.5001, -37.75) -> (-7.5001, -37.75)
  line L649 (-15.5001, -35.25) -> (-17.5001, -35.25)
  line L650 (-10.0001, -37.75) -> (-10.0001, -39.75)
  line L651 (-5.0001, -35.25) -> (-5.0001, -37.25)
  line L652 (-17.5001, -42.25) -> (-15.5001, -42.25)
  line L653 (-15.5001, -30.25) -> (-17.5001, -30.25)
  line L654 (-17.5001, -37.25) -> (-15.5001, -37.25)
  line L655 (-5.0001, -42.25) -> (-3.0001, -42.25)
  line L656 (-25.0001, -42.25) -> (-23.0001, -42.25)
  line L657 (-7.5001, -39.75) -> (-5.5001, -39.75)
  line L658 (-7.5001, -40.25) -> (-7.5001, -42.25)
  line L659 (-3.0001, -39.75) -> (-3.0001, -37.75)
  line L660 (-10.0001, -35.25) -> (-10.0001, -37.25)
  line L661 (-8.0001, -37.75) -> (-10.0001, -37.75)
  line L662 (-5.5001, -39.75) -> (-5.5001, -37.75)
  line L663 (-25.0001, -34.75) -> (-23.0001, -34.75)
  line L664 (-15.5001, -37.75) -> (-17.5001, -37.75)
  line L665 (-15.5001, -40.25) -> (-17.5001, -40.25)
  line L666 (-23.0001, -40.25) -> (-25.0001, -40.25)
  line L667 (-23.0001, -32.75) -> (-25.0001, -32.75)
  line L668 (-7.5001, -35.25) -> (-7.5001, -37.25)
  line L669 (-17.5001, -39.75) -> (-15.5001, -39.75)
  line L670 (-23.0001, -30.25) -> (-25.0001, -30.25)
  line L671 (-10.5001, -42.25) -> (-10.5001, -40.25)
  line L672 (-10.5001, -39.75) -> (-10.5001, -37.75)
  line L673 (-10.0001, -37.25) -> (-8.0001, -37.25)
  line L674 (-15.5001, -32.75) -> (-17.5001, -32.75)
  line L675 (-8.0001, -37.25) -> (-8.0001, -35.25)
  line L676 (-17.5001, -32.25) -> (-15.5001, -32.25)
  line L677 (-5.0001, -37.25) -> (-3.0001, -37.25)
  line L678 (-10.0001, -39.75) -> (-8.0001, -39.75)
  line L679 (-5.0001, -40.25) -> (-5.0001, -42.25)
  line L680 (-7.5001, -37.75) -> (-7.5001, -39.75)
  line L681 (-50.5001, -30.25) -> (-52.5001, -30.25)
  line L682 (-50.5001, -40.25) -> (-52.5001, -40.25)
  line L683 (-50.5001, -35.25) -> (-52.5001, -35.25)
  line L684 (-52.5001, -32.25) -> (-50.5001, -32.25)
  line L685 (-52.5001, -34.75) -> (-50.5001, -34.75)
  line L686 (-52.5001, -42.25) -> (-50.5001, -42.25)
  line L687 (-52.5001, -39.75) -> (-50.5001, -39.75)
  line L688 (-50.5001, -37.75) -> (-52.5001, -37.75)
  line L689 (-50.5001, -32.75) -> (-52.5001, -32.75)
  line L690 (-52.5001, -37.25) -> (-50.5001, -37.25)
  line L691 (-52.5001, -32.75) -> (-52.5001, -34.75)
  line L692 (-52.5001, -35.25) -> (-52.5001, -37.25)
  line L693 (-45.0001, -32.75) -> (-45.0001, -34.75)
  line L694 (-52.5001, -37.75) -> (-52.5001, -39.75)
  line L695 (-52.5001, -40.25) -> (-52.5001, -42.25)
  line L696 (-52.5001, -30.25) -> (-52.5001, -32.25)
  line L697 (-50.0001, -42.25) -> (-48.0001, -42.25)
  line L698 (-45.0001, -40.25) -> (-45.0001, -42.25)
  line L699 (-47.5001, -39.75) -> (-45.5001, -39.75)
  line L700 (-47.5001, -42.25) -> (-45.5001, -42.25)
  line L701 (-50.0001, -40.25) -> (-50.0001, -42.25)
  line L702 (-43.0001, -40.25) -> (-45.0001, -40.25)
  line L703 (-45.0001, -39.75) -> (-43.0001, -39.75)
  line L704 (-48.0001, -40.25) -> (-50.0001, -40.25)
  line L705 (-47.5001, -40.25) -> (-47.5001, -42.25)
  line L706 (-45.5001, -42.25) -> (-45.5001, -40.25)
  line L707 (-43.0001, -42.25) -> (-43.0001, -40.25)
  line L708 (-15.0001, -37.25) -> (-13.0001, -37.25)
  line L709 (-3.0001, -32.25) -> (-3.0001, -30.25)
  line L710 (-3.0001, -34.75) -> (-3.0001, -32.75)
  line L711 (-8.0001, -34.75) -> (-8.0001, -32.75)
  line L712 (-38.0001, -37.75) -> (-40.0001, -37.75)
  line L713 (-5.5001, -34.75) -> (-5.5001, -32.75)
  line L714 (-30.0001, -34.75) -> (-28.0001, -34.75)
  line L715 (-40.0001, -37.75) -> (-40.0001, -39.75)
  line L716 (-28.0001, -37.75) -> (-30.0001, -37.75)
  line L717 (-10.5001, -32.25) -> (-10.5001, -30.25)
  line L718 (-15.0001, -35.25) -> (-15.0001, -37.25)
  line L719 (-5.5001, -35.25) -> (-7.5001, -35.25)
  line L720 (-30.5001, -37.75) -> (-32.5001, -37.75)
  line L721 (-5.0001, -32.25) -> (-3.0001, -32.25)
  line L722 (-13.0001, -37.75) -> (-15.0001, -37.75)
  line L723 (-15.0001, -34.75) -> (-13.0001, -34.75)
  line L724 (-28.0001, -35.25) -> (-30.0001, -35.25)
  line L725 (-12.5001, -35.25) -> (-12.5001, -37.25)
  line L726 (-15.5001, -37.25) -> (-15.5001, -35.25)
  line L727 (-28.0001, -32.75) -> (-30.0001, -32.75)
  line L728 (-32.5001, -37.25) -> (-30.5001, -37.25)
  line L729 (-38.0001, -40.25) -> (-40.0001, -40.25)
  line L730 (-28.0001, -42.25) -> (-28.0001, -40.25)
  line L731 (-40.0001, -39.75) -> (-38.0001, -39.75)
  line L732 (-32.5001, -37.75) -> (-32.5001, -39.75)
  line L733 (-40.5001, -40.25) -> (-42.5001, -40.25)
  line L734 (-7.5001, -32.25) -> (-5.5001, -32.25)
  line L735 (-7.5001, -30.25) -> (-7.5001, -32.25)
  line L736 (-38.0001, -32.75) -> (-40.0001, -32.75)
  line L737 (-5.0001, -30.25) -> (-5.0001, -32.25)
  line L738 (-38.0001, -35.25) -> (-40.0001, -35.25)
  line L739 (-7.5001, -34.75) -> (-5.5001, -34.75)
  line L740 (-38.0001, -42.25) -> (-38.0001, -40.25)
  line L741 (-38.0001, -37.25) -> (-38.0001, -35.25)
  line L742 (-12.5001, -37.25) -> (-10.5001, -37.25)
  line L743 (-5.0001, -32.75) -> (-5.0001, -34.75)
  line L744 (-10.0001, -32.75) -> (-10.0001, -34.75)
  line L745 (-15.0001, -32.75) -> (-15.0001, -34.75)
  line L746 (-40.0001, -40.25) -> (-40.0001, -42.25)
  line L747 (-13.0001, -35.25) -> (-15.0001, -35.25)
  line L748 (-40.0001, -35.25) -> (-40.0001, -37.25)
  line L749 (-42.5001, -37.25) -> (-40.5001, -37.25)
  line L750 (-10.5001, -34.75) -> (-10.5001, -32.75)
  line L751 (-3.0001, -30.25) -> (-5.0001, -30.25)
  line L752 (-38.0001, -39.75) -> (-38.0001, -37.75)
  line L753 (-5.5001, -32.75) -> (-7.5001, -32.75)
  line L754 (-40.0001, -42.25) -> (-38.0001, -42.25)
  line L755 (-5.5001, -32.25) -> (-5.5001, -30.25)
  line L756 (-10.0001, -32.25) -> (-8.0001, -32.25)
  line L757 (-8.0001, -35.25) -> (-10.0001, -35.25)
  line L758 (-13.0001, -34.75) -> (-13.0001, -32.75)
  line L759 (-10.0001, -34.75) -> (-8.0001, -34.75)
  line L760 (-8.0001, -32.75) -> (-10.0001, -32.75)
  line L761 (-22.5001, -32.25) -> (-20.5001, -32.25)
  line L762 (-3.0001, -35.25) -> (-5.0001, -35.25)
  line L763 (-40.0001, -37.25) -> (-38.0001, -37.25)
  line L764 (-13.0001, -37.25) -> (-13.0001, -35.25)
  line L765 (-30.5001, -39.75) -> (-30.5001, -37.75)
  line L766 (-10.5001, -30.25) -> (-12.5001, -30.25)
  line L767 (-5.5001, -30.25) -> (-7.5001, -30.25)
  line L768 (-22.5001, -42.25) -> (-20.5001, -42.25)
  line L769 (-42.5001, -42.25) -> (-40.5001, -42.25)
  line L770 (-28.0001, -40.25) -> (-30.0001, -40.25)
  line L771 (-8.0001, -32.25) -> (-8.0001, -30.25)
  line L772 (-40.5001, -42.25) -> (-40.5001, -40.25)
  line L773 (-22.5001, -37.25) -> (-20.5001, -37.25)
  line L774 (-30.0001, -39.75) -> (-28.0001, -39.75)
  line L775 (-28.0001, -30.25) -> (-30.0001, -30.25)
  line L776 (-32.5001, -42.25) -> (-30.5001, -42.25)
  line L777 (-13.0001, -40.25) -> (-15.0001, -40.25)
  line L778 (-32.5001, -40.25) -> (-32.5001, -42.25)
  line L779 (-23.0001, -39.75) -> (-23.0001, -37.75)
  line L780 (-20.5001, -40.25) -> (-22.5001, -40.25)
  line L781 (-22.5001, -35.25) -> (-22.5001, -37.25)
  line L782 (-22.5001, -32.75) -> (-22.5001, -34.75)
  line L783 (-10.5001, -40.25) -> (-12.5001, -40.25)
  line L784 (-10.0001, -40.25) -> (-10.0001, -42.25)
  line L785 (-3.0001, -37.25) -> (-3.0001, -35.25)
  line L786 (-13.0001, -42.25) -> (-13.0001, -40.25)
  line L787 (-15.0001, -42.25) -> (-13.0001, -42.25)
  line L788 (-8.0001, -40.25) -> (-10.0001, -40.25)
  line L789 (-8.0001, -30.25) -> (-10.0001, -30.25)
  line L790 (-3.0001, -42.25) -> (-3.0001, -40.25)
  line L791 (-15.0001, -39.75) -> (-13.0001, -39.75)
  line L792 (-30.5001, -40.25) -> (-32.5001, -40.25)
  line L793 (-5.5001, -37.25) -> (-5.5001, -35.25)
  line L794 (-23.0001, -42.25) -> (-23.0001, -40.25)
  line L795 (-12.5001, -39.75) -> (-10.5001, -39.75)
  line L796 (-72.5001, -40.25) -> (-72.5001, -42.25)
  line L797 (-22.5001, -30.25) -> (-22.5001, -32.25)
  line L798 (-15.0001, -40.25) -> (-15.0001, -42.25)
  line L799 (-3.0001, -32.75) -> (-5.0001, -32.75)
  line L800 (-20.5001, -30.25) -> (-22.5001, -30.25)
  line L801 (-40.5001, -37.75) -> (-42.5001, -37.75)
  line L802 (-12.5001, -42.25) -> (-10.5001, -42.25)
  line L803 (-40.0001, -34.75) -> (-38.0001, -34.75)
  line L804 (-7.5001, -32.75) -> (-7.5001, -34.75)
  line L805 (-5.5001, -40.25) -> (-7.5001, -40.25)
  line L806 (-30.5001, -42.25) -> (-30.5001, -40.25)
  line L807 (-27.5001, -40.25) -> (-27.5001, -42.25)
  line L808 (-12.5001, -37.75) -> (-12.5001, -39.75)
  line L809 (-10.5001, -35.25) -> (-12.5001, -35.25)
  line L810 (-10.5001, -32.75) -> (-12.5001, -32.75)
  line L811 (-30.0001, -40.25) -> (-30.0001, -42.25)
  line L812 (-42.5001, -39.75) -> (-40.5001, -39.75)
  line L813 (-30.0001, -42.25) -> (-28.0001, -42.25)
  line L814 (-23.0001, -32.25) -> (-23.0001, -30.25)
  line L815 (-5.0001, -39.75) -> (-3.0001, -39.75)
  line L816 (-22.5001, -40.25) -> (-22.5001, -42.25)
  line L817 (-3.0001, -40.25) -> (-5.0001, -40.25)
  line L818 (-12.5001, -40.25) -> (-12.5001, -42.25)
  line L819 (-23.0001, -34.75) -> (-23.0001, -32.75)
  line L820 (-20.5001, -32.75) -> (-22.5001, -32.75)
  line L821 (-23.0001, -37.25) -> (-23.0001, -35.25)
  line L822 (-72.5001, -42.25) -> (-70.5001, -42.25)
  line L823 (-15.5001, -42.25) -> (-15.5001, -40.25)
  line L824 (-70.5001, -40.25) -> (-72.5001, -40.25)
  line L825 (-10.0001, -30.25) -> (-10.0001, -32.25)
  line L826 (-22.5001, -37.75) -> (-22.5001, -39.75)
  line L827 (-40.5001, -39.75) -> (-40.5001, -37.75)
  line L828 (-42.5001, -37.75) -> (-42.5001, -39.75)
  line L829 (-45.0001, -35.25) -> (-45.0001, -37.25)
  line L830 (-45.5001, -37.75) -> (-47.5001, -37.75)
  line L831 (-47.5001, -34.75) -> (-45.5001, -34.75)
  line L832 (-43.0001, -37.75) -> (-45.0001, -37.75)
  line L833 (-80.0001, -34.75) -> (-78.0001, -34.75)
  line L834 (-70.5001, -32.25) -> (-70.5001, -30.25)
  line L835 (-70.0001, -35.25) -> (-70.0001, -37.25)
  line L836 (-60.5001, -30.25) -> (-62.5001, -30.25)
  line L837 (-75.5001, -32.25) -> (-75.5001, -30.25)
  line L838 (-80.0001, -32.25) -> (-78.0001, -32.25)
  line L839 (-60.5001, -40.25) -> (-62.5001, -40.25)
  line L840 (-78.0001, -37.75) -> (-80.0001, -37.75)
  line L841 (-60.5001, -35.25) -> (-62.5001, -35.25)
  line L842 (-68.0001, -37.75) -> (-70.0001, -37.75)
  line L843 (-63.0001, -37.75) -> (-65.0001, -37.75)
  line L844 (-62.5001, -39.75) -> (-60.5001, -39.75)
  line L845 (-80.0001, -30.25) -> (-80.0001, -32.25)
  line L846 (-62.5001, -35.25) -> (-62.5001, -37.25)
  line L847 (-62.5001, -37.25) -> (-60.5001, -37.25)
  line L848 (-62.5001, -32.25) -> (-60.5001, -32.25)
  line L849 (-65.5001, -37.25) -> (-65.5001, -35.25)
  line L850 (-75.0001, -35.25) -> (-75.0001, -37.25)
  line L851 (-80.0001, -37.25) -> (-78.0001, -37.25)
  line L852 (-62.5001, -32.75) -> (-62.5001, -34.75)
  line L853 (-62.5001, -37.75) -> (-62.5001, -39.75)
  line L854 (-73.0001, -37.25) -> (-73.0001, -35.25)
  line L855 (-63.0001, -34.75) -> (-63.0001, -32.75)
  line L856 (-65.0001, -39.75) -> (-63.0001, -39.75)
  line L857 (-65.0001, -35.25) -> (-65.0001, -37.25)
  line L858 (-65.5001, -39.75) -> (-65.5001, -37.75)
  line L859 (-78.0001, -32.75) -> (-80.0001, -32.75)
  line L860 (-68.0001, -32.75) -> (-70.0001, -32.75)
  line L861 (-60.5001, -37.75) -> (-62.5001, -37.75)
  line L862 (-65.0001, -37.75) -> (-65.0001, -39.75)
  line L863 (-73.0001, -34.75) -> (-73.0001, -32.75)
  line L864 (-62.5001, -42.25) -> (-60.5001, -42.25)
  line L865 (-75.5001, -37.25) -> (-75.5001, -35.25)
  line L866 (-80.0001, -35.25) -> (-80.0001, -37.25)
  line L867 (-65.0001, -34.75) -> (-63.0001, -34.75)
  line L868 (-62.5001, -34.75) -> (-60.5001, -34.75)
  line L869 (-68.0001, -35.25) -> (-70.0001, -35.25)
  line L870 (-63.0001, -32.75) -> (-65.0001, -32.75)
  line L871 (-70.5001, -34.75) -> (-70.5001, -32.75)
  line L872 (-70.5001, -37.25) -> (-70.5001, -35.25)
  line L873 (-70.0001, -34.75) -> (-68.0001, -34.75)
  line L874 (-70.0001, -32.25) -> (-68.0001, -32.25)
  line L875 (-65.0001, -32.75) -> (-65.0001, -34.75)
  line L876 (-63.0001, -30.25) -> (-65.0001, -30.25)
  line L877 (-68.0001, -30.25) -> (-70.0001, -30.25)
  line L878 (-65.5001, -34.75) -> (-65.5001, -32.75)
  line L879 (-63.0001, -35.25) -> (-65.0001, -35.25)
  line L880 (-65.5001, -32.25) -> (-65.5001, -30.25)
  line L881 (-63.0001, -37.25) -> (-63.0001, -35.25)
  line L882 (-78.0001, -30.25) -> (-80.0001, -30.25)
  line L883 (-63.0001, -39.75) -> (-63.0001, -37.75)
  line L884 (-65.0001, -37.25) -> (-63.0001, -37.25)